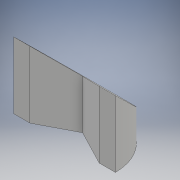
# Autodesk Inventor part: Part3
Saved by Autodesk Inventor 2018 (Build 220112000, 112)
## iProperties
Created: 2017-11-15
Part Number: Part3
Material: Generic
Document SubType Name: Modeling
Designer: kurti
Density: 1 g/cm^3
Appearance: Default
Author: kurti
Autodesk Inventor part; units mm, degrees
ref_plane "YZ Plane" through (0, 0, 0) normal (1, 0, 0) x (0, 1, 0)
ref_plane "XZ Plane" through (0, 0, 0) normal (0, 1, 0) x (-1, 0, 0)
ref_plane "XY Plane" through (0, 0, 0) normal (0, 0, 1) x (1, 0, 0)
sketch "Sketch1" plane through (0, 0, 0) normal (1, 0, 0) x (0, 1, 0)
  line L0 (0, 0) -> (0, -9.25)
  line L1 (0, 0) -> (0, 9.25)
  line L2 (0, -9.25) -> (14.25, -9.25)
  line L3 (14.25, -9.25) -> (14.25, -4.75)
  line L4 (14.25, -4.75) -> (0, 9.25)
  dimension "d0" = 9.25
  dimension "d1" = 9.25
  dimension "d2" = 14.25
  dimension "d3" = 4.5
  constraints: 10 end point, 2 vertical, 1 horizontal, 1 perpendicular
  measures "d0" distance of L0.start L0.end
  measures "d1" distance of L0.start L1.end
  measures "d2" distance of L0.end L2.end
  measures "d3" distance of L2.end L3.end
sketch "Sketch2" plane through (0, 0, 0) normal (0, 0, 1) x (1, 0, 0)
  line L0 (0, 0) -> (14.125, 0) construction
  line L1 (0, 0) -> (-14.125, 0) construction
  line L2 (-14.125, 0) -> (-9.625, 0)
  line L3 (14.125, 0) -> (9.625, 0)
  arc A0 (14.125, 0) -> (-14.125, 0) centre (0, 0) ccw
  line L4 (0, 0) -> (0, 5) construction
  line L5 (-9.625, 0) -> (0, 5)
  line L6 (0, 5) -> (9.625, 0)
  line L7 (-25, 30) -> (25, 30)
  line L8 (25, 30) -> (25, -20)
  line L9 (25, -20) -> (-25, -20)
  line L10 (-25, -20) -> (-25, 30)
  line L11 (-25, 30) -> (25, -20) construction
  line L12 (25, 30) -> (-25, -20) construction
  dimension "d6" = 4.5
  dimension "d7" = 4.5
  dimension "d8" = 14.125
  dimension "d9" = 5
  dimension "d12" = 50
  dimension "d13" = 50
  constraints: 26 end point, 3 horizontal, 2 midpoint, 2 parallel, 2 point on circle, 2 point on line, 1 centre point, 1 coincident, 1 perpendicular, 1 vertical
  measures "d6" distance of L1.end L2.end
  measures "d7" distance of L0.end L3.end
  measures "d8" distance of L0.start L1.end
  measures "d9" distance of L4.start L4.end
  measures "d12" distance of L7.start L7.end
  measures "d13" distance of L7.end L8.end
extrude "Extrusion1" add sketch "Sketch1" along normal mid plane 28.25
extrude "Extrusion2" cut sketch "Sketch2" along normal mid plane 28.25
equation "\"d1\" = d0"
equation "\"d10\" = 2 * d8"
equation "\"d14\" = 2 * d8"
body "Solid1"
